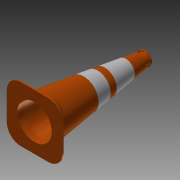
# Autodesk Inventor part: 36 inch
Saved by Autodesk Inventor 2015 (Build 190159000, 159)
## iProperties
Created: 2018-01-10
Part Number: 36 inch
Material: ABS Plastic
Document SubType Name: Modeling
Designer: Syamsi
Density: 1.06 g/cm^3
Appearance: Smooth - Light Orange
Author: Syamsi
Autodesk Inventor part; units mm, degrees
ref_plane "YZ Plane" through (0, 0, 0) normal (1, 0, 0) x (0, 1, 0)
ref_plane "XZ Plane" through (0, 0, 0) normal (0, 1, 0) x (-1, 0, 0)
ref_plane "XY Plane" through (0, 0, 0) normal (0, 0, 1) x (1, 0, 0)
sketch "Sketch2" plane through (0, 0, 0) normal (0, 0, 1) x (1, 0, 0)
  line L0 (0, 0) -> (0, 711.2) construction
  line L1 (0, 681.2) -> (-30, 681.2)
  line L2 (-30, 681.2) -> (-30, 711.2)
  line L3 (-30, 711.2) -> (-50, 711.2)
  line L4 (-50, 711.2) -> (-64.2857, 609.6)
  line L5 (-64.2857, 609.6) -> (-85.7143, 457.2) construction
  line L6 (-85.7143, 457.2) -> (-92.8571, 406.4)
  line L7 (-92.8571, 406.4) -> (-107.1429, 304.8) construction
  line L8 (-107.1429, 304.8) -> (-150, 0)
  line L9 (-150, 0) -> (0, 0) construction
  line L10 (-107.1429, 304.8) -> (-108.1331, 304.9392)
  line L11 (-108.1331, 304.9392) -> (-93.8474, 406.5392)
  line L12 (-93.8474, 406.5392) -> (-92.8571, 406.4)
  line L13 (-86.7045, 457.3392) -> (-65.276, 609.7392)
  line L14 (-65.276, 609.7392) -> (-64.2857, 609.6)
  line L15 (-85.7143, 457.2) -> (-86.7045, 457.3392)
  line L16 (0, 656.2) -> (-32.4875, 656.2)
  line L17 (-32.4875, 656.2) -> (-124.7541, 0)
  line L18 (-150, 0) -> (-124.7541, 0)
  line L19 (0, 681.2) -> (0, 656.2)
  dimension "d0" = 711.2
  dimension "d1" = 101.6
  dimension "d2" = 152.4
  dimension "d3" = 50.8
  dimension "d4" = 101.6
  dimension "d5" = 711.2
  dimension "d6" = 20
  dimension "d7" = 30
  dimension "d8" = 30
  dimension "d9" = 150
  dimension "d10" = 1
  dimension "d11" = 1
  dimension "d13" = 25
  dimension "d14" = 25
  constraints: 40 end point, 8 point on line, 7 perpendicular, 3 parallel, 2 collinear, 1 horizontal, 1 vertical
  measures "d0" distance of L0.start L0.end
  measures "d1" vertical distance of L3.end L4.end
  measures "d2" vertical distance of L4.end L5.end
  measures "d3" vertical distance of L5.end L6.end
  measures "d4" vertical distance of L6.end L7.end
  measures "d5" distance between parallel lines of L9 L3
  measures "d6" distance of L2.end L3.end
  measures "d7" distance of L1.start L1.end
  measures "d8" distance of L0.end L1.start
  measures "d9" distance of L0.start L8.end
  measures "d10" distance of L7.end L10.end
  measures "d11" distance of L5.end L15.end
  measures "d13" distance between parallel lines of L4 L17
  measures "d14" distance between parallel lines of L1 L16
revolve "Revolution1" add sketch "Sketch2" angle 360 about axis through (0, 0, 0) along (0, 1, 0)
sketch "Sketch3" plane through (0, 0, 0) normal (1, 0, 0) x (0, 1, 0)
  line L0 (0, 0) -> (711.2, 0)
  line L1 (711.2, -30) -> (711.2, 30) projected
  line L2 (711.2, -50) -> (711.2, 50) projected
  line L3 (711.2, -30) -> (751.2, -30)
  line L4 (751.2, -30) -> (751.2, -50)
  line L5 (751.2, -50) -> (739.1998, -50)
  line L6 (739.1998, -50) -> (739.1998, -40)
  line L7 (739.1998, -40) -> (711.2, -40)
  line L8 (711.2, -30) -> (711.2, -40)
  dimension "d16" = 711.2
  dimension "d17" = 40
  dimension "d18" = 10
  dimension "d19" = 10
  dimension "d20" = 12.0002
  constraints: 14 end point, 4 perpendicular, 1 collinear, 1 horizontal, 1 midpoint, 1 point on line
  measures "d16" distance of L0.start L0.end
  measures "d17" distance of L1.start L3.end
  measures "d18" distance between parallel lines of L3 L7
  measures "d19" distance of L5.end L6.end
  measures "d20" distance of L4.end L5.end
revolve "Revolution2" add sketch "Sketch3" angle 360 about axis through (0, 0, 0) along (0, 1, 0)
fillet "Fillet1" radius 4 5 edges at (50, 711.2, 0) (0, 711.2, 40) (0, 739.1998, 40) (0, 739.1998, 50) (0, 751.2, 50)
sketch "Sketch4" plane through (0, 0, 0) normal (0, -1, 0) x (1, 0, 0)
  line L0 (-200, 200) -> (200, 200)
  line L1 (200, 200) -> (200, -200)
  line L2 (200, -200) -> (-200, -200)
  line L3 (-200, -200) -> (-200, 200)
  line L4 (-200, 200) -> (200, -200) construction
  line L5 (200, 200) -> (-200, -200) construction
  point P0 (0, 0)
  dimension "d23" = 400
  dimension "d24" = 400
  constraints: 12 end point, 2 midpoint, 2 parallel, 1 horizontal, 1 perpendicular
  measures "d23" distance of L1.end L2.end
  measures "d24" distance of L0.end L1.end
extrude "Extrusion1" add sketch "Sketch4" along normal blind 50
sketch "Sketch5" plane through (0, -50, 0) normal (0, -1, 0) x (1, 0, 0)
  circle A0 centre (0, 0) radius 124.7541 projected
extrude "Extrusion2" cut sketch "Sketch5" against normal blind 50
fillet "Fillet2" radius 100 4 edges at (200, -25, -200) (200, -25, 200) (-200, -25, 200) (-200, -25, -200)
chamfer "Chamfer1" distance 40 distance2 40 4 edges at (200, 0, 0) (0, 0, -200) (-200, 0, 0) (0, 0, 200) measured on face at (183.2518, 0, 2.8544)
equation "\"d5\" = d0"
equation "\"d14\" = d13"
equation "\"d23\" = d24"
body "Solid1"
